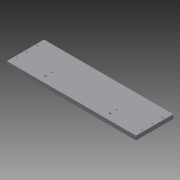
# Autodesk Inventor part: licht_2m
Saved by Autodesk Inventor 2015 (Build 190159000, 159)
## iProperties
Created: 2018-01-11
Part Number: licht_2m
Material: Generisch
Document SubType Name: Modeling
Designer: schueler
Density: 1 g/cm^3
Appearance: Vorgabe
Author: schueler
Autodesk Inventor part; units mm, degrees
ref_plane "YZ Plane" through (0, 0, 0) normal (1, 0, 0) x (0, 1, 0)
ref_plane "XZ Plane" through (0, 0, 0) normal (0, 1, 0) x (-1, 0, 0)
ref_plane "XY Plane" through (0, 0, 0) normal (0, 0, 1) x (1, 0, 0)
sketch "Skizze1" plane through (0, 0, 0) normal (0, 0, 1) x (1, 0, 0)
  line L0 (0, 0) -> (500, 0)
  line L1 (500, 0) -> (500, 144)
  line L2 (500, 144) -> (0, 144)
  line L3 (0, 144) -> (0, 0)
  line L4 (0, 25) -> (500, 25) construction
  line L5 (0, 50) -> (500, 50) construction
  line L6 (250, 0) -> (250, 144) construction
  line L7 (125, 0) -> (125, 144) construction
  line L8 (375, 144) -> (375, 0) construction
  circle A0 centre (125, 50) radius 2.5
  circle A1 centre (375, 50) radius 2.5
  circle A2 centre (375, 25) radius 3.5
  circle A3 centre (125, 25) radius 3.5
  line L9 (492, 144) -> (492, 0) construction
  line L10 (500, 112) -> (0, 112) construction
  line L11 (500, 32) -> (0, 32) construction
  circle A4 centre (492, 112) radius 1.5
  circle A5 centre (492, 32) radius 1.5
  line L12 (8, 144) -> (8, 0) construction
  circle A6 centre (8, 112) radius 1.5
  circle A7 centre (8, 72) radius 1.5
  circle A8 centre (8, 32) radius 1.5
  circle A9 centre (492, 72) radius 1.5
  point P0 (-875, 50)
  point P1 (-875, 25)
  point P2 (500, 72)
  dimension "d0" = 500
  dimension "d1" = 144
  dimension "d2" = 25
  dimension "d3" = 50
  dimension "d4" = 125
  dimension "d5" = 125
  dimension "d9" = 5
  dimension "d10" = 5
  dimension "d13" = 7
  dimension "d14" = 7
  dimension "d20" = 8
  dimension "d21" = 40
  dimension "d22" = 40
  dimension "d23" = 3
  dimension "d24" = 3
  dimension "d25" = 8
  dimension "d26" = 3
  dimension "d27" = 3
  dimension "d28" = 3
  dimension "d29" = 3
  constraints: 34 point on line, 26 end point, 10 centre point, 8 perpendicular, 5 midpoint, 3 parallel, 1 horizontal
  measures "d0" distance of L2.end L1.end
  measures "d1" distance of L1.end L0.end
  measures "d2" distance of L0.end L4.end
  measures "d3" distance of L0.end L5.end
  measures "d4" distance of L8.start L6.end
  measures "d5" distance of L7.end L6.end
  measures "d9" diameter of A0
  measures "d10" diameter of A1
  measures "d13" diameter of A2
  measures "d14" diameter of A3
  measures "d20" distance of L1.end L9.start
  measures "d21" distance of L10.start point (500, 72)
  measures "d22" distance of L11.start point (500, 72)
  measures "d23" diameter of A4
  measures "d24" diameter of A5
  measures "d25" distance of L12.start L2.end
  measures "d26" diameter of A6
  measures "d27" diameter of A7
  measures "d28" diameter of A8
  measures "d29" diameter of A9
extrude "Extrusion1" add sketch "Skizze1" along normal blind 16
hole "Bohrung1" at (375, 25, 0) at (125, 25, 0) at (-875, 25, 0) direction (0, 0, 1) diameter 10 depth 12 tip angle 118
hole "Bohrung4" at (375, 50, 0) at (125, 50, 0) direction (0, 0, 1) diameter 7 depth 12 tip angle 118
sketch "Skizze2" plane through (0, 0, 16) normal (0, 0, 1) x (1, 0, 0)
  circle A0 centre (250, 72) radius 1.5 projected
  circle A1 centre (492, 112) radius 1.5 projected
  circle A2 centre (492, 72) radius 1.5 projected
  circle A3 centre (492, 32) radius 1.5 projected
  circle A4 centre (8, 72) radius 1.5 projected
  circle A5 centre (8, 112) radius 1.5 projected
  circle A6 centre (8, 32) radius 1.5 projected
  circle A7 centre (250, 32) radius 1.5 projected
  circle A8 centre (250, 112) radius 1.5 projected
  point P0 (0, 0)
hole "Bohrung7" at (492, 112, 16) at (492, 72, 16) at (492, 32, 16) at (8, 72, 16) at (8, 32, 16) at (8, 112, 16) direction (0, 0, -1) diameter 3 depth 8 countersink diameter 8 countersink angle 90
sketch "Skizze3" plane through (0, 144, 0) normal (0, 1, 0) x (1, 0, 0)
  line L0 (500, -16) -> (0, -16) construction
  line L1 (0, -16) -> (0, 0) construction
  line L2 (0, 0) -> (500, 0) construction
  line L3 (500, 0) -> (500, -16) construction
  line L4 (500, -8) -> (0, -8) construction
  line L5 (0, 0) -> (0, -16) construction
  line L6 (0, -16) -> (500, -16) construction
  line L7 (460, -16) -> (460, 0) construction
  line L8 (0, 0) -> (500, 0) construction
  line L9 (40, -16) -> (40, 0) construction
  line L10 (250, -16) -> (250, 0) construction
  point P0 (460, -8)
  point P1 (250, -8)
  point P2 (40, -8)
  dimension "d120" = 40
  dimension "d121" = 40
  constraints: 16 end point, 7 midpoint, 4 point on line, 3 parallel, 2 perpendicular, 1 horizontal
  measures "d120" distance of L7.start L0.start
  measures "d121" distance of L9.start L0.end
hole "Bohrung12" at (460, 144, 8) at (250, 144, 8) at (40, 144, 8) direction (0, -1, 0) diameter 3 depth 30 tip angle 118
